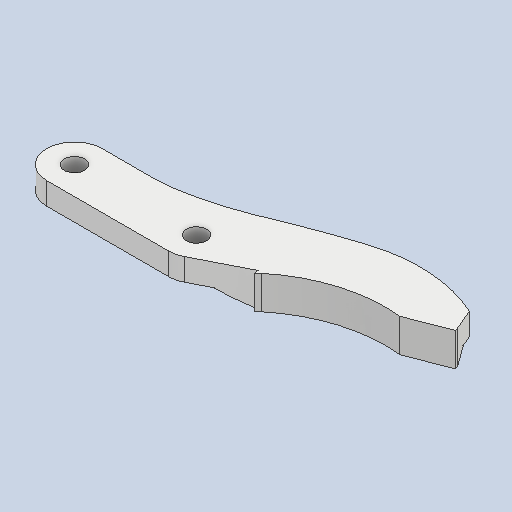
# Autodesk Inventor part: lapak2
Saved by Autodesk Inventor 2023 (Build 270158000, 158)
## iProperties
Part Number: lapak2
Material: ABS Plastic
Document SubType Name: Modeling
Designer: denyh
Density: 1.06 g/cm^3
Appearance: Smooth - White
Mass: 2.80888 g
Surface Area: 20.4393 cm^2
Volume: 2.64989 cm^3
Author: denyh
Autodesk Inventor part; units mm, degrees
ref_plane "YZ Plane" through (0, 0, 0) normal (1, 0, 0) x (0, 1, 0)
ref_plane "XZ Plane" through (0, 0, 0) normal (0, 1, 0) x (-1, 0, 0)
ref_plane "XY Plane" through (0, 0, 0) normal (0, 0, 1) x (1, 0, 0)
sketch "Náčrt1" plane through (0, 0, 0) normal (0, 0, 1) x (1, 0, 0)
  circle A0 centre (0, 0) radius 1.825
  circle A1 centre (22, 0) radius 1.825
  arc A2 (0, 5) -> (0, -5) centre (0, 0) ccw
  line L0 (0, 0) -> (-0.516, 0)
  line L1 (0, 5) -> (8.645, 5)
  arc A3 (8.645, 5) -> (13.8862, 5.4744) centre (8.645, 34.19) ccw
  arc A4 (8.645, 5) -> (8.645, 5) centre (6.8603, 48.5893) ccw
  arc A5 (58.5138, 12.7037) -> (38.8579, 13.8954) centre (47.1549, -11.9507) ccw
  line L2 (22, -5) -> (0, -5)
  line L3 (24.2622, -4.459) -> (33.0865, 0.0179)
  line L4 (22, 0) -> (22, 6.29)
  line L5 (58.5138, 12.7037) -> (60.0748, 9.0208)
  arc A6 (52.9531, 6.2627) -> (33.0865, 0.0179) centre (50.3132, -20.062) ccw
  arc A7 (22, -5) -> (24.2622, -4.459) centre (22, 0) ccw
  line L6 (52.9531, 6.2627) -> (60.0748, 9.0208)
  line L7 (23.9587, 8.3506) -> (22.7174, 7.8453)
  arc A8 (38.8579, 13.8954) -> (23.9587, 8.3506) centre (92.1034, -151.9688) ccw
  arc A9 (13.8862, 5.4744) -> (23.9587, 8.3506) centre (4.237, 58.3407) ccw
  dimension "d0" = 3.65
  dimension "d2" = 3.65
  dimension "d3" = 10
  dimension "d8" = 0.516
  dimension "d17" = 9.895
  dimension "d18" = 63.1
  dimension "d19" = 20.825
  dimension "d21" = 4
  constraints: 16 end point, 16 point on circle, 10 centre point, 7 tangent, 3 coincident, 1 horizontal, 1 vertical
  measures "d0" diameter of A0
  measures "d2" diameter of A1
  measures "d3" diameter of A2
  measures "d8" distance of L0.start L0.end
  measures "d17" distance of L3.start L3.end
  measures "d18" angle of L3 L4
  measures "d19" distance of L3.end L6.start
  measures "d21" distance of L5.start L5.end
extrude "Vysunutí1" add sketch "Náčrt1" along normal blind 4 contours L1 A4 A3 A9 A8 A5 L5 L6 A6 L3 A7 L2 A2 | L1 A4 picked at (7.0586, 4.9892)
sketch "Náčrt7" plane through (0, 0, 0) normal (0, 0, -1) x (-1, 0, 0)
  arc A0 (-33.0865, 0.0179) -> (-52.9531, 6.2627) centre (-50.3132, -20.062) ccw projected
  line L0 (-60.0748, 9.0208) -> (-52.9531, 6.2627) projected
  line L1 (-60.2916, 8.4611) -> (-53.047, 5.6554) projected
  arc A1 (-33.8826, -0.0897) -> (-53.047, 5.6554) centre (-50.3132, -20.062) ccw projected
  line L2 (-33.2047, -0.6673) -> (-33.0865, 0.0179)
  line L3 (-33.8826, -0.0897) -> (-33.2047, -0.6673) projected
  line L4 (-59.2939, 10.8632) -> (-60.0748, 9.0208) projected
  line L5 (-60.2916, 8.4611) -> (-60.0748, 9.0208)
  point P0 (0, 0)
  constraints: 4 end point
extrude "Vysunutí5" add sketch "Náčrt7" along normal blind 2 and the other way blind 4
chamfer "Zkosení3" distance 2 angle 45 2 edges at (42.3795, 5.1772, 0) (56.514, 7.6418, 0)
